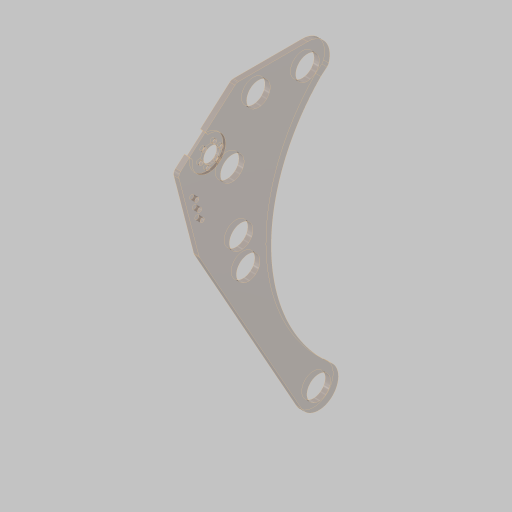
# Autodesk Inventor part: GP4-008
Saved by Autodesk Inventor 2023.5 (Build 275446000, 446)
## iProperties
Created: 2025-01-28
Part Number: GP4-008
Material: Polycarbonate, Smoke
Document SubType Name: Modeling
Designer: slick
Density: 1.2 g/cm^3
Appearance: Polycarbonate - Smoked
Mass: 208.631 g
Surface Area: 668.483 cm^2
Volume: 173.859 cm^3
Author: slick
Autodesk Inventor part; units mm, degrees
ref_plane "YZ Plane" through (0, 0, 0) normal (1, 0, 0) x (0, 1, 0)
ref_plane "XZ Plane" through (0, 0, 0) normal (0, 1, 0) x (-1, 0, 0)
ref_plane "XY Plane" through (0, 0, 0) normal (0, 0, 1) x (1, 0, 0)
sketch "Sketch1" plane through (0, 0, 0) normal (1, 0, 0) x (0, 1, 0)
  circle A0 centre (0, 0) radius 203.2 construction
  circle A1 centre (165.1, 167.1631) radius 38.1 construction
  circle A2 centre (165.1, 167.1631) radius 31.75 construction
  circle A3 centre (-177.8, 153.586) radius 38.1 construction
  circle A4 centre (-177.8, 153.586) radius 31.75 construction
  circle A5 centre (279.4, 30.6697) radius 38.1 construction
  circle A6 centre (279.4, 30.6697) radius 31.75 construction
  line L0 (371.6722, 159.6086) -> (293.9242, 243.3925) construction
  line L1 (293.9242, 243.3925) -> (72.8278, 38.2242) construction
  line L2 (72.8278, 38.2242) -> (150.5758, -45.5597) construction
  line L3 (150.5758, -45.5597) -> (371.6722, 159.6086) construction
  line L4 (371.6722, 159.6086) -> (72.8278, 38.2242) construction
  line L5 (293.9242, 243.3925) -> (150.5758, -45.5597) construction
  line L6 (165.1, 167.1631) -> (279.4, 30.6697) construction
  point P0 (222.25, 98.9164)
  dimension "d0" = 406.4
  dimension "d1" = 76.2
  dimension "d2" = 6.35
  dimension "d4" = 114.3
  dimension "d5" = 301.625
  dimension "d6" = 177.8
  dimension "d51" = 165.1
  dimension "d52" = 279.4
  dimension "d53" = 30.6697
  constraints: 14 end point, 7 centre point, 4 equal radius, 4 tangent, 3 midpoint, 2 coincident, 2 parallel, 1 perpendicular
  measures "d0" diameter of A0
  measures "d1" diameter of A1
  measures "d2" radial gap between concentric circles of A1 A2
  measures "d4" distance of L2.end L1.end
  measures "d5" distance of L1.end L0.end
  measures "d6" horizontal distance of A3.centre point (0, 0)
  measures "d51" horizontal distance of point (0, 0) L6.start
  measures "d52" horizontal distance of point (0, 0) L6.end
  measures "d53" vertical distance of point (0, 0) L6.end
sketch "Sketch4" plane through (0, 0, 0) normal (1, 0, 0) x (0, 1, 0)
  circle A0 centre (0, 0) radius 203.2 construction
  circle A1 centre (165.1, 167.1631) radius 38.1 construction
  circle A2 centre (165.1, 167.1631) radius 31.75 construction
  circle A3 centre (-177.8, 153.586) radius 38.1 construction
  circle A4 centre (-177.8, 153.586) radius 31.75 construction
  circle A5 centre (279.4, 30.6697) radius 38.1 construction
  circle A6 centre (279.4, 30.6697) radius 31.75 construction
  line L0 (371.6722, 159.6086) -> (293.9242, 243.3925) construction
  line L1 (293.9242, 243.3925) -> (72.8278, 38.2242) construction
  line L2 (72.8278, 38.2242) -> (150.5758, -45.5597) construction
  line L3 (150.5758, -45.5597) -> (371.6722, 159.6086) construction
  line L4 (371.6722, 159.6086) -> (72.8278, 38.2242) construction
  line L5 (293.9242, 243.3925) -> (150.5758, -45.5597) construction
  line L6 (165.1, 167.1631) -> (279.4, 30.6697) construction
  circle A7 centre (-177.8, 153.586) radius 14.2875
  circle A8 centre (165.1, 167.1631) radius 14.2875
  circle A9 centre (279.4, 30.6697) radius 14.2875
  circle A10 centre (165.1, 167.1631) radius 23.8125 construction
  circle A11 centre (279.4, 30.6697) radius 23.8125 construction
  circle A12 centre (-177.8, 153.586) radius 23.8125 construction
  line L7 (261.1433, 15.3815) -> (146.8433, 151.8749)
  line L8 (309.92, 115.3835) -> (248.7672, 188.4102)
  line L9 (309.92, 115.3835) -> (303.1398, 28.8105)
  line L10 (248.7672, 188.4102) -> (130.1238, 323.85)
  line L11 (130.1238, 323.85) -> (31.75, 298.45)
  line L12 (31.75, 298.45) -> (-189.4509, 174.3536)
  arc A13 (148.3669, 150.2209) -> (-159.7797, 138.0199) centre (0, 0) ccw
  arc A14 (148.3669, 150.2209) -> (146.8433, 151.8749) centre (165.1, 167.1631) ccw
  arc A15 (256.4562, 24.2964) -> (303.1398, 28.8105) centre (279.4, 30.6697) ccw
  line L13 (332.7982, 201.5005) -> (111.7018, -3.6678) construction
  arc A16 (-189.4509, 174.3536) -> (-159.7797, 138.0199) centre (-177.8, 153.586) ccw
  point P0 (222.25, 98.9164)
  point P1 (279.3436, 151.8969)
  point P2 (261.1433, 15.3815)
  point P3 (147.5854, 150.9888)
  dimension "d27" = 28.575
  dimension "d29" = 9.525
  dimension "d31" = 101.6
  dimension "d33" = 101.6
  dimension "d35" = 95.25
  dimension "d58" = 298.45
  dimension "d59" = 323.85
  dimension "d60" = 31.75
  constraints: 15 end point, 15 point on circle, 10 centre point, 7 coincident, 5 equal radius, 5 tangent, 3 midpoint, 1 parallel, 1 point on line
  measures "d27" diameter of A7
  measures "d29" radial gap between concentric circles of A9 A11
  measures "d31" distance between parallel lines of L7 L8
  measures "d33" distance of L10.end L11.end
  measures "d35" distance of L8.start L8.end
  measures "d58" vertical distance of point (0, 0) L11.end
  measures "d59" vertical distance of point (0, 0) L10.end
  measures "d60" horizontal distance of point (0, 0) L11.end
extrude "Extrusion2" add sketch "Sketch4" along normal blind 6.35 contours L7 A14 A13 | L7 A13 A16 L12 L11 L10 L8 L9 A15
sketch "Sketch5" plane through (6.35, 0, 0) normal (1, 0, 0) x (0, 0, -1)
  line L0 (-323.85, 130.1238) -> (-298.45, 31.75) projected
  line L1 (-301.2085, 93.2336) -> (-294.8585, 68.6402) construction
  point P0 (0, 0)
  point P1 (-298.0335, 80.9369)
  point P2 (-311.15, 80.9369)
  point P3 (-298.0335, 80.9369)
  point P4 (-311.15, 80.9369)
  dimension "d39" = 12.7
  dimension "d57" = 25.4
  constraints: 3 midpoint, 2 end point, 1 coincident, 1 horizontal alignment, 1 parallel
  measures "d39" distance from line of L0 L1.start
  measures "d57" distance of L1.start L1.end
hole "Hole2" at (6.35, 93.2336, 301.2085) at (6.35, 80.9369, 298.0335) at (6.35, 68.6402, 294.8585) direction (-1, 0, 0) diameter 5.1054 end through all clearance for "Flat Head Machine Screw (82)" size "#10" standard "Ansi Unified Screw Threads"
sketch "Sketch6" plane through (6.35, 0, 0) normal (1, 0, 0) x (0, 0, -1)
  circle A0 centre (-298.0335, 80.9369) radius 2.5527 projected
  circle A1 centre (-301.2085, 93.2336) radius 2.5527 projected
  circle A2 centre (-294.8585, 68.6402) radius 2.5527 projected
  arc A3 (-15.3815, 261.1433) -> (-28.8105, 303.1398) centre (-30.6697, 279.4) ccw projected
  line L0 (-28.8105, 303.1398) -> (-115.3835, 309.92) projected
  line L1 (-115.3835, 309.92) -> (-188.4102, 248.7672) projected
  line L2 (-188.4102, 248.7672) -> (-323.85, 130.1238) projected
  line L3 (-323.85, 130.1238) -> (-298.45, 31.75) projected
  line L4 (-298.45, 31.75) -> (-174.3536, -189.4509) projected
  arc A4 (-174.3536, -189.4509) -> (-138.0199, -159.7797) centre (-153.586, -177.8) ccw projected
  arc A5 (-150.9888, 147.5854) -> (-138.0199, -159.7797) centre (0, 0) ccw projected
  line L5 (-150.9888, 147.5854) -> (-15.3815, 261.1433) projected
  circle A6 centre (-30.6697, 279.4) radius 14.2875 projected
  circle A7 centre (-167.1631, 165.1) radius 14.2875 projected
  circle A8 centre (-153.586, -177.8) radius 14.2875 projected
  circle A9 centre (-167.1631, 165.1) radius 26.9875 construction
  line L6 (-167.1631, 192.0875) -> (-253.1141, 192.0875)
  line L7 (-188.4102, 248.7672) -> (-323.85, 130.1238) construction
  circle A10 centre (-167.1631, 165.1) radius 14.2875 construction
  line L8 (-150.9888, 147.5854) -> (-15.3815, 261.1433) construction
  arc A11 (-142.138, 154.997) -> (-167.1631, 192.0875) centre (-167.1631, 165.1) ccw
  dimension "d65" = 12.7
  constraints: 4 point on circle, 2 centre point, 2 end point, 2 point on line, 1 coincident, 1 horizontal, 1 tangent
  measures "d65" radial gap between concentric circles of A7 A9
extrude "Extrusion3" cut sketch "Sketch6" against normal blind 25.4 contours A0 | A1 | A2 | L5 A11 L6 L2 L1 L0 A3 | A8
fillet "Fillet1" radius 6.604 4 edges at (3.175, 192.0875, 253.1141) (3.175, 130.1238, 323.85) (3.175, 31.75, 298.45) (3.175, 154.997, 142.138)
sketch "Sketch8" plane through (6.35, 0, 0) normal (1, 0, 0) x (0, 0, -1)
  circle A0 centre (-283.6185, 131.5988) radius 7.6454 construction
  circle A1 centre (-283.6185, 131.5988) radius 19.05 construction
  circle A2 centre (-167.1631, 165.1) radius 28.6512 construction
  arc A3 (-320.7904, 132.804) -> (-322.8331, 126.1854) centre (-316.4388, 127.8364) ccw construction
  line L0 (-320.7904, 132.804) -> (-254.9821, 190.4511) construction
  arc A4 (-250.6306, 192.0875) -> (-254.9821, 190.4511) centre (-250.6306, 185.4835) ccw construction
  line L1 (-250.6306, 192.0875) -> (-167.1631, 192.0875) construction
  arc A5 (-141.4456, 156.9185) -> (-167.1631, 192.0875) centre (-167.1631, 165.1) ccw construction
  arc A6 (-143.4989, 153.8574) -> (-141.4456, 156.9185) centre (-147.7388, 158.9206) ccw construction
  line L2 (-143.4989, 153.8574) -> (-150.9888, 147.5854) construction
  arc A7 (-150.9888, 147.5854) -> (-138.0199, -159.7797) centre (0, 0) ccw construction
  arc A8 (-174.3536, -189.4509) -> (-138.0199, -159.7797) centre (-153.586, -177.8) ccw construction
  line L3 (-174.3536, -189.4509) -> (-298.0299, 31.0012) construction
  arc A9 (-298.6647, 32.5814) -> (-298.0299, 31.0012) centre (-292.2704, 34.2324) ccw construction
  line L4 (-298.6647, 32.5814) -> (-322.8331, 126.1854) construction
  circle A10 centre (-298.0335, 80.9369) radius 2.5527 construction
  circle A11 centre (-301.2085, 93.2336) radius 2.5527 construction
  circle A12 centre (-294.8585, 68.6402) radius 2.5527 construction
  circle A13 centre (-153.586, -177.8) radius 14.2875 construction
  circle A14 centre (-167.1631, 165.1) radius 14.2875 construction
  circle A15 centre (-283.6185, 131.5988) radius 9.525
  circle A16 centre (-167.1631, 165.1) radius 14.2875
  circle A17 centre (-247.5393, 27.9128) radius 14.2875
  circle A18 centre (-247.5393, 27.9128) radius 19.05 construction
  circle A19 centre (-239.0544, -9.2303) radius 19.05 construction
  circle A20 centre (-239.0544, -9.2303) radius 14.2875
  dimension "d76" = 15.2908
  dimension "d77" = 38.1
  dimension "d78" = 57.3024
  dimension "d79" = 121.1783
  dimension "d81" = 25.4
  dimension "d83" = 19.05
  dimension "d84" = 28.575
  dimension "d85" = 158.9989
  dimension "d87" = 38.1
  dimension "d88" = 188.9989
  dimension "d111" = 31.75
  constraints: 9 centre point, 6 coincident, 4 equal radius
  measures "d76" diameter of A0
  measures "d77" diameter of A1
  measures "d78" diameter of A2
  measures "d79" distance of A2.centre A0.centre
  measures "d81" distance from line of A0.centre L0
  measures "d83" diameter of A15
  measures "d84" diameter of A16
  measures "d85" distance of A17.centre A2.centre
  measures "d87" diameter of A18
  measures "d88" distance of A13.centre A19.centre
  measures "d111" distance from line of L3 A19.centre
extrude "Extrusion4" cut sketch "Sketch8" against normal through all
sketch "Sketch11" plane through (0, 0, 0) normal (-1, 0, 0) x (0, 0, 1)
  circle A0 centre (247.5393, 27.9128) radius 14.2875 construction
  circle A1 centre (283.6185, 131.5988) radius 9.525 construction
  circle A2 centre (239.0544, -9.2303) radius 14.2875 construction
  arc A3 (322.8331, 126.1854) -> (320.7904, 132.804) centre (316.4388, 127.8364) ccw construction
  line L0 (322.8331, 126.1854) -> (298.6647, 32.5814) construction
  arc A4 (298.0299, 31.0012) -> (298.6647, 32.5814) centre (292.2704, 34.2324) ccw construction
  line L1 (298.0299, 31.0012) -> (174.3536, -189.4509) construction
  arc A5 (138.0199, -159.7797) -> (174.3536, -189.4509) centre (153.586, -177.8) ccw construction
  arc A6 (138.0199, -159.7797) -> (150.9888, 147.5854) centre (0, 0) ccw construction
  line L2 (150.9888, 147.5854) -> (143.4989, 153.8574) construction
  arc A7 (141.4456, 156.9185) -> (143.4989, 153.8574) centre (147.7388, 158.9206) ccw construction
  arc A8 (167.1631, 192.0875) -> (141.4456, 156.9185) centre (167.1631, 165.1) ccw construction
  line L3 (167.1631, 192.0875) -> (250.6306, 192.0875) construction
  arc A9 (254.9821, 190.4511) -> (250.6306, 192.0875) centre (250.6306, 185.4835) ccw construction
  line L4 (254.9821, 190.4511) -> (320.7904, 132.804) construction
  circle A10 centre (298.0335, 80.9369) radius 2.5527 construction
  circle A11 centre (301.2085, 93.2336) radius 2.5527 construction
  circle A12 centre (294.8585, 68.6402) radius 2.5527 construction
  circle A13 centre (153.586, -177.8) radius 14.2875 construction
  circle A14 centre (167.1631, 165.1) radius 14.2875 construction
  circle A15 centre (283.6185, 131.5988) radius 20.32
  line L5 (284.5175, 151.8989) -> (290.8021, 159.0733)
  line L6 (303.6236, 135.1623) -> (309.9082, 142.3366)
  line L7 (309.9082, 142.3366) -> (290.8021, 159.0733)
  line L8 (254.9821, 190.4511) -> (320.7904, 132.804) construction
  line L9 (283.6185, 131.5988) -> (300.3551, 150.7049) construction
  dimension "d112" = 40.64
  dimension "d113" = 25.4
  constraints: 8 end point, 4 point on line, 3 perpendicular, 2 point on circle, 1 centre point, 1 coincident, 1 midpoint
  measures "d112" diameter of A15
  measures "d113" distance between parallel lines of L6 L5
extrude "Extrusion6" cut sketch "Sketch11" against normal blind 3.175
sketch "Sketch12" plane through (3.175, 0, 0) normal (-1, 0, 0) x (0, 0, 1)
  circle A0 centre (247.5393, 27.9128) radius 14.2875 construction
  circle A1 centre (283.6185, 131.5988) radius 9.525 construction
  circle A2 centre (239.0544, -9.2303) radius 14.2875 construction
  arc A3 (322.8331, 126.1854) -> (320.7904, 132.804) centre (316.4388, 127.8364) ccw construction
  line L0 (322.8331, 126.1854) -> (298.6647, 32.5814) construction
  arc A4 (298.0299, 31.0012) -> (298.6647, 32.5814) centre (292.2704, 34.2324) ccw construction
  line L1 (298.0299, 31.0012) -> (174.3536, -189.4509) construction
  arc A5 (138.0199, -159.7797) -> (174.3536, -189.4509) centre (153.586, -177.8) ccw construction
  arc A6 (138.0199, -159.7797) -> (150.9888, 147.5854) centre (0, 0) ccw construction
  line L2 (150.9888, 147.5854) -> (143.4989, 153.8574) construction
  arc A7 (141.4456, 156.9185) -> (143.4989, 153.8574) centre (147.7388, 158.9206) ccw construction
  arc A8 (167.1631, 192.0875) -> (141.4456, 156.9185) centre (167.1631, 165.1) ccw construction
  line L3 (167.1631, 192.0875) -> (250.6306, 192.0875) construction
  arc A9 (254.9821, 190.4511) -> (250.6306, 192.0875) centre (250.6306, 185.4835) ccw construction
  line L4 (254.9821, 190.4511) -> (290.8021, 159.0733) construction
  line L5 (290.8021, 159.0733) -> (309.9082, 142.3366) construction
  line L6 (309.9082, 142.3366) -> (320.7904, 132.804) construction
  line L7 (290.8021, 159.0733) -> (284.5175, 151.8989) construction
  arc A10 (284.5175, 151.8989) -> (303.6236, 135.1623) centre (283.6185, 131.5988) ccw construction
  line L8 (303.6236, 135.1623) -> (309.9082, 142.3366) construction
  circle A11 centre (298.0335, 80.9369) radius 2.5527 construction
  circle A12 centre (301.2085, 93.2336) radius 2.5527 construction
  circle A13 centre (294.8585, 68.6402) radius 2.5527 construction
  circle A14 centre (153.586, -177.8) radius 14.2875 construction
  circle A15 centre (167.1631, 165.1) radius 14.2875 construction
  circle A16 centre (247.5393, 27.9128) radius 14.2875 construction
  circle A17 centre (283.6185, 131.5988) radius 9.525 construction
  circle A18 centre (239.0544, -9.2303) radius 14.2875 construction
  arc A19 (322.8331, 126.1854) -> (320.7904, 132.804) centre (316.4388, 127.8364) ccw construction
  line L9 (322.8331, 126.1854) -> (298.6647, 32.5814) construction
  arc A20 (298.0299, 31.0012) -> (298.6647, 32.5814) centre (292.2704, 34.2324) ccw construction
  line L10 (298.0299, 31.0012) -> (174.3536, -189.4509) construction
  arc A21 (138.0199, -159.7797) -> (174.3536, -189.4509) centre (153.586, -177.8) ccw construction
  arc A22 (138.0199, -159.7797) -> (150.9888, 147.5854) centre (0, 0) ccw construction
  line L11 (150.9888, 147.5854) -> (143.4989, 153.8574) construction
  arc A23 (141.4456, 156.9185) -> (143.4989, 153.8574) centre (147.7388, 158.9206) ccw construction
  arc A24 (167.1631, 192.0875) -> (141.4456, 156.9185) centre (167.1631, 165.1) ccw construction
  line L12 (167.1631, 192.0875) -> (250.6306, 192.0875) construction
  arc A25 (254.9821, 190.4511) -> (250.6306, 192.0875) centre (250.6306, 185.4835) ccw construction
  line L13 (254.9821, 190.4511) -> (290.8021, 159.0733) construction
  line L14 (290.8021, 159.0733) -> (309.9082, 142.3366) construction
  line L15 (309.9082, 142.3366) -> (320.7904, 132.804) construction
  line L16 (290.8021, 159.0733) -> (284.5175, 151.8989) construction
  arc A26 (284.5175, 151.8989) -> (303.6236, 135.1623) centre (283.6185, 131.5988) ccw construction
  line L17 (303.6236, 135.1623) -> (309.9082, 142.3366) construction
  circle A27 centre (298.0335, 80.9369) radius 2.5527 construction
  circle A28 centre (301.2085, 93.2336) radius 2.5527 construction
  circle A29 centre (294.8585, 68.6402) radius 2.5527 construction
  circle A30 centre (153.586, -177.8) radius 14.2875 construction
  circle A31 centre (167.1631, 165.1) radius 14.2875 construction
  circle A32 centre (283.6185, 131.5988) radius 12.7 construction
  point P0 (279.5294, 143.6226)
  point P1 (271.1611, 134.0695)
  point P2 (275.2501, 122.0458)
  point P3 (287.7075, 119.5751)
  point P4 (296.0758, 129.1282)
  point P5 (291.9868, 141.1519)
  dimension "d116" = 25.4
  dimension "d117" = 19.05
  dimension "d120" = 360
  constraints: 1 coincident, 10 other
  measures "d117" distance from line of L5 point (279.529, 143.623)
hole "Hole5" at (3.175, 143.6226, 279.5294) at (3.175, 134.0695, 271.1611) at (3.175, 122.0458, 275.2501) at (3.175, 119.5751, 287.7075) at (3.175, 129.1282, 296.0758) at (3.175, 141.1519, 291.9868) direction (1, 0, 0) diameter 5.1054 end through all clearance for "Flat Head Machine Screw (82)" size "#10" standard "Ansi Unified Screw Threads"
sketch "Sketch13" plane through (6.35, 0, 0) normal (1, 0, 0) x (0, 0, -1)
  circle A0 centre (-296.0758, 129.1282) radius 2.5527 construction
  circle A1 centre (-275.2501, 122.0458) radius 2.5527 construction
  circle A2 centre (-279.5294, 143.6226) radius 2.5527 construction
  circle A3 centre (-271.1611, 134.0695) radius 2.5527 construction
  circle A4 centre (-287.7075, 119.5751) radius 2.5527 construction
  circle A5 centre (-291.9868, 141.1519) radius 2.5527 construction
  circle A6 centre (-247.5393, 27.9128) radius 14.2875 construction
  circle A7 centre (-283.6185, 131.5988) radius 9.525 construction
  circle A8 centre (-239.0544, -9.2303) radius 14.2875 construction
  arc A9 (-320.7904, 132.804) -> (-322.8331, 126.1854) centre (-316.4388, 127.8364) ccw construction
  line L0 (-320.7904, 132.804) -> (-254.9821, 190.4511) construction
  arc A10 (-250.6306, 192.0875) -> (-254.9821, 190.4511) centre (-250.6306, 185.4835) ccw construction
  line L1 (-250.6306, 192.0875) -> (-167.1631, 192.0875) construction
  arc A11 (-141.4456, 156.9185) -> (-167.1631, 192.0875) centre (-167.1631, 165.1) ccw construction
  arc A12 (-143.4989, 153.8574) -> (-141.4456, 156.9185) centre (-147.7388, 158.9206) ccw construction
  line L2 (-143.4989, 153.8574) -> (-150.9888, 147.5854) construction
  arc A13 (-150.9888, 147.5854) -> (-138.0199, -159.7797) centre (0, 0) ccw construction
  arc A14 (-174.3536, -189.4509) -> (-138.0199, -159.7797) centre (-153.586, -177.8) ccw construction
  line L3 (-174.3536, -189.4509) -> (-298.0299, 31.0012) construction
  arc A15 (-298.6647, 32.5814) -> (-298.0299, 31.0012) centre (-292.2704, 34.2324) ccw construction
  line L4 (-298.6647, 32.5814) -> (-322.8331, 126.1854) construction
  circle A16 centre (-298.0335, 80.9369) radius 2.5527 construction
  circle A17 centre (-301.2085, 93.2336) radius 2.5527 construction
  circle A18 centre (-294.8585, 68.6402) radius 2.5527 construction
  circle A19 centre (-153.586, -177.8) radius 14.2875 construction
  circle A20 centre (-167.1631, 165.1) radius 14.2875 construction
  circle A21 centre (-226.6273, 167.1472) radius 14.2875
  circle A22 centre (-226.6273, 167.1472) radius 23.749 construction
  circle A23 centre (-167.1631, 165.1) radius 35.7505 construction
  circle A24 centre (-283.6185, 131.5988) radius 6.35 construction
  circle A25 centre (-258.3004, 104.8511) radius 30.48 construction
  circle A26 centre (-258.3004, 104.8511) radius 14.2875
  circle A27 centre (-226.6273, 167.1472) radius 30.5054 construction
  dimension "d133" = 28.575
  dimension "d134" = 47.498
  dimension "d135" = 71.501
  dimension "d138" = 12.7
  dimension "d139" = 60.96
  dimension "d142" = 69.8856
  dimension "d143" = 61.0108
  dimension "d144" = 57.15
  constraints: 7 centre point, 5 coincident, 2 tangent, 1 equal radius
  measures "d133" diameter of A21
  measures "d134" diameter of A22
  measures "d135" diameter of A23
  measures "d138" diameter of A24
  measures "d139" diameter of A25
  measures "d142" distance of A25.centre A21.centre
  measures "d143" diameter of A27
  measures "d144" distance from line of L4 A25.centre
extrude "Extrusion7" cut sketch "Sketch13" against normal through all
body "Solid2"
